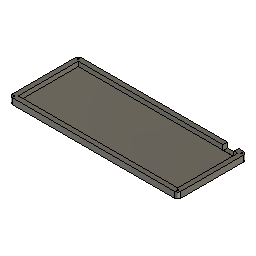
bottom (Autodesk Fusion 360 design; units mm, degrees)
part number: 2026-03-14-13-55-50-480
Autodesk Fusion 360 part; units mm, degrees
sketch "Sketch1" plane through (0, 0, 0) normal (0, 0, 1) x (1, 0, 0)
  line L0 (-221.214, 50) -> (125, 50)
  line L1 (125, 50) -> (125, -80.212)
  line L2 (125, -80.212) -> (-221.214, -80.212)
  line L3 (-221.214, -80.212) -> (-221.214, 50)
  line L4 (-231.214, 60) -> (135, 60)
  line L5 (135, 60) -> (135, -90.212)
  line L6 (135, -90.212) -> (-231.214, -90.212)
  line L7 (-231.214, -90.212) -> (-231.214, 60)
  circle A0 centre (-225.714, 54.5) radius 1.45
  circle A1 centre (129.5, 54.5) radius 1.45
  circle A2 centre (129.5, -84.712) radius 1.45
  circle A3 centre (-225.714, -84.712) radius 1.45
  dimension "d1" = 130.212
  dimension "d2" = 346.214
  dimension "d3" = 10
  dimension "d4" = 10
  dimension "d5" = 10
  dimension "d6" = 10
  dimension "d15" = 2.9
  dimension "d16" = 5.5
  dimension "d17" = 5.5
  dimension "d18" = 2.9
  dimension "d19" = 5.5
  dimension "d20" = 5.5
  dimension "d21" = 2.9
  dimension "d22" = 5.5
  dimension "d23" = 5.5
  dimension "d24" = 2.9
  dimension "d25" = 5.5
  dimension "d26" = 5.5
  constraint horizontal L0
  constraint vertical L1
  constraint horizontal L2
  constraint vertical L3
  constraint horizontal L4
  constraint vertical L5
  constraint horizontal L6
  constraint vertical L7
  measures "d1" distance of L0 L2
  measures "d2" distance of L1 L3
  measures "d3" distance of L0 L4
  measures "d4" distance of L1 L5
  measures "d5" distance of L2 L6
  measures "d6" distance of L3 L7
  measures "d15" diameter of A0
  measures "d16" distance of L4 A0.centre
  measures "d17" distance of L7 A0.centre
  measures "d18" diameter of A1
  measures "d19" distance of L5 A1.centre
  measures "d20" distance of L4 A1.centre
  measures "d21" diameter of A2
  measures "d22" distance of L5 A2.centre
  measures "d23" distance of L6 A2.centre
  measures "d24" diameter of A3
  measures "d25" distance of L6 A3.centre
  measures "d26" distance of L7 A3.centre
extrude "Extrude1" add sketch "Sketch1" along normal blind 3 contours L0 L1 L2 L3
extrude "Extrude2" add sketch "Sketch1" along normal blind 13 contours L4 L5 L6 L7 | A0 | A1 | A2 | A3
sketch "Sketch3" plane through (0, 60, 0) normal (0, 1, 0) x (-1, 0, 0)
  line L0 (-135, 0) -> (231.214, 0)
  line L1 (231.214, 0) -> (231.214, 13)
  line L2 (231.214, 13) -> (-135, 13)
  line L3 (-135, 13) -> (-135, 0)
  line L4 (-117.016, 13) -> (-93.016, 13)
  line L5 (-93.016, 13) -> (-93.016, 2)
  line L6 (-93.016, 2) -> (-117.016, 2)
  line L7 (-117.016, 2) -> (-117.016, 13)
  dimension "d11" = 24
  dimension "d12" = 17.984
  constraint horizontal L4
  constraint vertical L5
  constraint horizontal L6
  constraint vertical L7
  constraint coincident L2 L4.start
  measures "d11" distance of L4.start L4.end
  measures "d12" distance of L3 L7
extrude "Extrude3" cut sketch "Sketch3" against normal blind 10 contours L2 L4 L5 L6 L7
extrude "Extrude4" cut sketch "Sketch1" along normal blind 13 contours A0 | A1 | A2 | A3
fillet "Fillet1" radius 7 4 edges at (135, -90.212, 6.5) (135, 60, 6.5) (-231.214, 60, 6.5) (-231.214, -90.212, 6.5)
